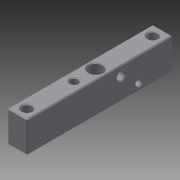
# Autodesk Inventor part: Upper Die Center Support
Saved by Autodesk Inventor 2015 (Build 190159000, 159)
## iProperties
Created: 2018-04-03
Part Number: Upper Die Center Support
Material: Generic
Document SubType Name: Modeling
Designer: Administrator
Density: 1 g/cm^3
Appearance: Default
Author: Administrator
Autodesk Inventor part; units mm, degrees
ref_plane "YZ Plane" through (0, 0, 0) normal (1, 0, 0) x (0, 1, 0)
ref_plane "XZ Plane" through (0, 0, 0) normal (0, 1, 0) x (-1, 0, 0)
ref_plane "XY Plane" through (0, 0, 0) normal (0, 0, 1) x (1, 0, 0)
sketch "Sketch1" plane through (0, 0, 0) normal (0, 0, 1) x (1, 0, 0)
  line L0 (0, 0) -> (15.875, 0)
  line L1 (15.875, 0) -> (15.875, 25.4)
  line L2 (15.875, 25.4) -> (0, 25.4)
  line L3 (0, 25.4) -> (0, 0)
  dimension "d0" = 15.875
  dimension "d1" = 25.4
  constraints: 8 end point, 2 parallel, 1 horizontal, 1 perpendicular
  measures "d0" distance of L1.end L2.end
  measures "d1" distance of L0.end L1.end
extrude "Extrusion1" add sketch "Sketch1" along normal blind 117.475
chamfer "Chamfer1" distance 0.762 angle 45 11 edges at (15.875, 25.4, 58.7375) (7.9375, 25.4, 117.475) (0, 25.4, 58.7375) (7.9375, 25.4, 0) (15.875, 12.7, 0) (15.875, 0, 58.7375) (0, 12.7, 0) (0, 0, 58.7375) (15.875, 12.7, 117.475) (0, 12.7, 117.475) (7.9375, 0, 117.475)
sketch "Sketch2" plane through (0.762, 25.4, 0.762) normal (0, 1, 0) x (1, 0, 0)
  line L0 (14.351, 0.762) -> (0, 0.762) projected
  line L1 (0, -116.713) -> (14.351, -116.713) projected
  line L2 (-0.762, 0) -> (-0.762, -115.951) projected
  line L3 (15.113, -115.951) -> (15.113, 0) projected
  circle A0 centre (7.1755, -108.7755) radius 3.9688
  circle A1 centre (7.1755, -70.6755) radius 3.175
  circle A2 centre (7.1755, -53.213) radius 5.5563
  circle A3 centre (7.1755, -7.1755) radius 3.9688
  point P0 (-0.762, 0.762)
  dimension "d7" = 7.9375
  dimension "d8" = 7.9375
  dimension "d9" = 71.4375
  dimension "d10" = 53.975
  dimension "d11" = 7.9375
  dimension "d12" = 7.9375
  dimension "d13" = 6.35
  dimension "d14" = 11.1125
  dimension "d15" = 7.9375
  constraints: 4 centre point, 4 coincident
  measures "d7" distance from line of L1 point (7.176, -108.776)
  measures "d8" distance from line of point (7.176, -108.776) L3
  measures "d9" distance from line of L0 point (7.176, -70.675)
  measures "d10" distance from line of point (7.176, -53.213) L0
  measures "d11" distance from line of L0 point (7.176, -7.175)
  measures "d12" diameter of A0
  measures "d13" diameter of A1
  measures "d14" diameter of A2
  measures "d15" diameter of A3
extrude "Extrusion2" cut sketch "Sketch2" against normal blind 117.475
sketch "Sketch3" plane through (15.875, 0.762, 0.762) normal (1, 0, 0) x (0, 0, -1)
  line L0 (0.762, -0.762) -> (0.762, 23.876) projected
  line L1 (-115.951, -0.762) -> (0.762, -0.762) projected
  circle A0 centre (-40.513, 16.7005) radius 3.175
  circle A1 centre (-26.2255, 4.8006) radius 2.3813
  dimension "d18" = 26.9875
  dimension "d19" = 5.5626
  dimension "d20" = 17.4625
  dimension "d21" = 41.275
  dimension "d22" = 6.35
  dimension "d23" = 4.7625
  constraints: 2 centre point, 2 coincident
  measures "d18" distance from line of L0 point (-26.226, 4.801)
  measures "d19" distance from line of point (-26.226, 4.801) L1
  measures "d20" distance from line of L1 point (-40.513, 16.701)
  measures "d21" distance from line of L0 point (-40.513, 16.701)
  measures "d22" diameter of A0
  measures "d23" diameter of A1
extrude "Extrusion3" cut sketch "Sketch3" against normal blind 117.475
chamfer "Chamfer2" distance 0.762 angle 45 11 edges at (2.3812, 25.4, 53.975) (4.7625, 25.4, 71.4375) (3.9687, 25.4, 109.5375) (3.9687, 25.4, 7.9375) (15.875, 17.4625, 44.45) (15.875, 5.5626, 29.3688) (7.9375, 0, 0) (3.9687, 0, 7.9375) (2.3812, 0, 53.975) (4.7625, 0, 71.4375) (3.9687, 0, 109.5375)
body "Solid1"
